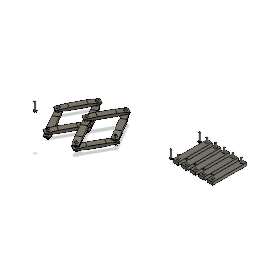
Collapse model encube (Autodesk Fusion 360 design; units mm, degrees)
Autodesk Fusion 360 part; units mm, degrees
sketch "Sketch6" plane through (0, 0, 0) normal (0, 1, 0) x (1, 0, 0)
  line L0 (20, 40) -> (40, 40)
  line L1 (40, 40) -> (40, -80)
  line L2 (40, -80) -> (20, -80)
  line L3 (20, -80) -> (20, 40)
  circle A0 centre (30, -70) radius 5
  circle A1 centre (30, 30) radius 5
  circle A2 centre (30, 30) radius 3.5
  dimension "d15" = 20
  dimension "d16" = 120
  dimension "d17" = 10
  dimension "d18" = 10
  dimension "d19" = 7
  measures "d17" diameter of A0
  measures "d18" diameter of A1
  measures "d19" diameter of A2
extrude "Extrude4" add sketch "Sketch6" along normal blind 10 makes body 1 at (33.4956, 6.6667, -29.8255) makes body 2 at (38.2593, 0, 3.8246)
extrude "Extrude5" add 1 faces at (30.1843, 10, -30.3192) along direction (0, 1, 0) blind 15 on bodies 1 bodies 1
extrude "Extrude6" add 1 faces at (29.8594, 0, -31.0235) along direction (0, -1, 0) blind 2 on bodies 1 bodies 1
sketch "Sketch7" plane through (0, -2, 0) normal (0, -1, 0) x (1, 0, 0)
  circle A0 centre (30, -30) radius 3.5
  circle A1 centre (30, -30) radius 5.5
  dimension "d27" = 11
  measures "d27" diameter of A1
extrude "Extrude7" add sketch "Sketch7" along normal blind 2 contours A0 | A1 bodies 1
copy_body "CopyPasteBodies1" bodies 1 makes body 3
move_body "Move1" bodies 3 to x (1, 0, 0) y (0, 1, 0) z (0, 0, 1) at (0, -1.5, 100)
copy_body "CopyPasteBodies2" bodies 2 3 1 makes body 4 makes body 5 makes body 6
move_body "Move2" bodies 4 5 6 to x (1, 0, 0) y (0, 1, 0) z (0, 0, 1) at (10, -5, 0)
move_body "Move3" bodies 4 5 6 to x (1, 0, 0) y (0, 1, 0) z (0, 0, 1) at (25, 0, 0)
copy_body "CopyPasteBodies3" bodies 6 4 5 makes body 7 makes body 8 makes body 9
move_body "Move4" bodies 7 8 9 to x (1, 0, 0) y (0, 1, 0) z (0, 0, 1) at (10, -5, 0)
move_body "Move5" bodies 4 5 6 to x (1, 0, 0) y (0, 1, 0) z (0, 0, 1) at (-10, 4.9138, 0)
move_body "Move6" bodies 8 7 9 to x (1, 0, 0) y (0, 1, 0) z (0, 0, 1) at (9.3387, 10, 3.5763)
copy_body "CopyPasteBodies4" bodies 9 8 7 makes body 10 makes body 11 makes body 12
move_body "Move7" bodies 10 11 12 to x (1, 0, 0) y (0, 1, 0) z (0, 0, 1) at (30, 0, 0)
copy_body "CopyPasteBodies5" bodies 11 12 10 makes body 13 makes body 14 makes body 15
move_body "Move8" bodies 13 14 15 to x (1, 0, 0) y (0, 1, 0) z (0, 0, 1) at (30, 0, 0)
copy_body "CopyPasteBodies6" bodies 11 12 10 makes body 16 makes body 17 makes body 18
move_body "Move9" bodies 16 17 18 to x (1, 0, 0) y (0, 1, 0) z (0, 0, 1) at (60, 0, 0)
copy_body "CopyPasteBodies7" bodies 11 12 10 makes body 19 makes body 20 makes body 21
move_body "Move10" bodies 19 20 21 to x (1, 0, 0) y (0, 1, 0) z (0, 0, 1) at (-110, 0, 0)
copy_body "CopyPasteBodies8" bodies 11 12 10 makes body 22 makes body 23 makes body 24
move_body "Move11" bodies 22 23 24 to x (1, 0, 0) y (0, 1, 0) z (0, 0, 1) at (90, 0, 0)
move_body "Move12" bodies 19 20 21 to x (0.866025, 0, -0.5) y (0, 1, 0) z (0.5, 0, 0.866025) at (17.4534, 0, -7.7105)
move_body "Move13" bodies 3 1 2 to x (0.866025, 0, 0.5) y (0, 1, 0) z (-0.5, 0, 0.866025) at (35.5324, 0, -103.6086)
move_body "Move14" bodies 3 2 1 to x (1, 0, 0) y (0, 1, 0) z (0, 0, 1) at (-18.3852, 0, -5.657)
move_body "Move15" bodies 20 to x (1, 0, 0) y (0, 1, 0) z (0, 0, 1) at (-36.4098, 0, 16.5628)
move_body "Move16" bodies 2 to x (1, 0, 0) y (0, 1, 0) z (0, 0, 1) at (0, 12, 0)
move_body "Move17" bodies 16 5 6 11 4 23 24 22 12 13 10 18 7 8 14 15 17 9 to x (1, 0, 0) y (0, 1, 0) z (0, 0, 1) at (120, 0, -170)
copy_body "CopyPasteBodies9" bodies 19 2 3 21 1 makes body 25 makes body 26 makes body 27 makes body 28 makes body 29
move_body "Move18" bodies 25 26 27 28 29 to x (-1, 0, 0) y (0, 1, 0) z (0, 0, -1) at (58.6773, 0, -92.8475)
move_body "Move19" bodies 25 27 26 29 28 to x (1, 0, 0) y (0, 1, 0) z (0, 0, 1) at (80, 0, 0)
move_body "Move20" bodies 29 to x (1, 0, 0) y (0, 1, 0) z (0, 0, 1) at (0, 125.2332, 92.6165)
move_body "Move21" bodies 28 to x (1, 0, 0) y (0, 1, 0) z (0, 0, 1) at (0, 145.8501, 251.9169)
move_body "Move22" bodies 27 26 25 to x (0.999848, 0, -0.017452) y (0, 1, 0) z (0.017452, 0, 0.999848) at (-22.4315, -0.8556, 27.9376)
move_body "Move23" bodies 4 to x (1, 0, 0) y (0, 1, 0) z (0, 0, 1) at (-67.9353, -2.2693, 166.4645)
move_body "Move24" bodies 4 to x (0.866025, 0, -0.5) y (0, 1, 0) z (0.5, 0, 0.866025) at (34.7719, 0, 42.6997)
move_body "Move25" bodies 4 to x (1, 0, 0) y (0, 1, 0) z (0, 0, 1) at (17, 0, 0)
move_body "Move26" bodies 4 to x (1, 0, 0) y (0, 1, 0) z (0, 0, 1) at (-20.6603, 15, 6.3397)
move_body "Move27" bodies 4 to x (1, 0, 0) y (0, 1, 0) z (0, 0, 1) at (0, 10, 0)
chamfer "Chamfer1" distance 35 angle 5 1 edges at (102.0647, 32.6444, -42.1957) measured on face at (147.3736, 32.6444, 19.7117) on bodies 4
chamfer "Chamfer2" distance 35 angle 5 1 edges at (102.0647, 22.6444, -42.1957) measured on face at (131.1298, 22.6444, -8.3722) on bodies 4
chamfer "Chamfer3" distance 35 angle 5 2 edges at (111.9128, 21.1444, -42.2817) (111.9128, 11.1444, -42.2817) measured on face at (83.4649, 21.1444, -8.0492) measured on face at (83.4649, 11.1444, -8.0492) on bodies 26
chamfer "Chamfer4" distance 35 angle 5 2 edges at (112.3288, 9.1444, -25.8462) (112.3288, -0.8556, -25.8462) measured on face at (65.9464, 9.1444, -86.9535) measured on face at (65.9464, -0.8556, -86.9535) on bodies 25
chamfer "Chamfer5" distance 35 angle 5 4 edges at (62.9989, 10, 62.4993) (62.9989, 0, 62.4993) (53.7357, 21.1444, 62.6727) (53.7357, 11.1444, 62.6727) measured on face at (33.9579, 10, 28.7686) measured on face at (33.9579, 0, 28.7686) measured on face at (83.5211, 21.1444, 8.6815) measured on face at (83.5211, 11.1444, 8.6815) on bodies 19 26
chamfer "Chamfer6" distance 35 angle 5 4 edges at (2.9989, 10, -41.4237) (2.9989, 0, -41.4237) (3.128, 22, -24.9836) (3.128, 12, -24.9836) measured on face at (33.9378, 10, 11.9148) measured on face at (33.9378, 0, 11.9148) measured on face at (32.169, 22, -58.7143) measured on face at (32.169, 12, -58.7143) on bodies 2 19
chamfer "Chamfer7" distance 35 angle 5 7 edges at (162.0647, 32.6444, 61.7273) (162.0647, 22.6444, 61.7273) (50.5242, 9.1444, -128.7063) (59.0959, 4.1444, -133.8567) (50.5242, -0.8556, -128.7063) (63.128, 22, -128.9066) (63.128, 12, -128.9066) measured on face at (131.3416, 32.6444, 8.2642) measured on face at (131.3416, 22.6444, 8.2642) measured on face at (82.3893, 9.1444, -75.9158) measured on face at (73.6887, 5.8111, -109.5703) measured on face at (82.3893, -0.8556, -75.9158) measured on face at (32.1891, 22, -75.568) measured on face at (32.1891, 12, -75.568) on bodies 2 4 25
move_body "Move28" bodies 21 to x (1, 0, 0) y (0, 1, 0) z (0, 0, 1) at (0, 0, 40)
move_body "Move29" bodies 1 to x (1, 0, 0) y (0, 1, 0) z (0, 0, 1) at (8.3083, 0, -18.1926)
move_body "Move30" bodies 3 to x (1, 0, 0) y (0, 1, 0) z (0, 0, 1) at (-40.9334, 0, -18.6937)
move_body "Move31" bodies 2 to x (0.999391, 0, -0.034899) y (0, 1, 0) z (0.034899, 0, 0.999391) at (2.2194, 0, 1.2079)
move_body "Move32" bodies 1 to x (1, 0, 0) y (0, 1, 0) z (0, 0, 1) at (-5.6261, -6.0621, 8.6157)
move_body "Move33" bodies 1 to x (1, 0, 0) y (0, 1, 0) z (0, 0, 1) at (-5, 0, 9)
move_body "Move34" bodies 1 to x (1, 0, 0) y (0, 1, 0) z (0, 0, 1) at (0.1223, 0, 0.2727)
move_body "Move35" bodies 1 to x (1, 0, 0) y (0, 1, 0) z (0, 0, 1) at (0, 5, 0)
move_body "Move36" bodies 3 to x (1, 0, 0) y (0, 1, 0) z (0, 0, 1) at (41.5864, 0, 19.2805)
extrude "Extrude8" add 1 faces at (106.7267, 22.6444, -32.702) along direction (0, 1, 0) blind 15 on bodies 27 bodies 27
copy_body "CopyPasteBodies10" bodies 26 makes body 30
move_body "Move37" bodies 30 to x (1, 0, 0) y (0, 1, 0) z (0, 0, 1) at (48.481, 0, -87.462)
move_body "Move38" bodies 30 to x (1, 0, 0) y (0, 1, 0) z (0, 0, 1) at (0, 22, 0)
copy_body "CopyPasteBodies11" bodies 26 makes body 31
move_body "Move39" bodies 31 to x (1, 0, 0) y (0, 1, 0) z (0, 0, 1) at (98.5603, 0, -0.7582)
move_body "Move40" bodies 21 to x (1, 0, 0) y (0, 1, 0) z (0, 0, 1) at (0.3864, 0, -39.9909)
move_body "Move41" bodies 28 to x (1, 0, 0) y (0, 1, 0) z (0, 0, 1) at (76.5599, -133.5476, -51.9802)
move_body "Move42" bodies 5 24 18 16 15 12 7 14 10 13 11 23 6 22 17 8 9 to x (1, 0, 0) y (0, 1, 0) z (0, 0, 1) at (160, 0, 0)
copy_body "CopyPasteBodies12" bodies 25 makes body 32
move_body "Move43" bodies 32 to x (0.999962, 0, 0.008727) y (0, 1, 0) z (-0.008727, 0, 0.999962) at (99.3452, 23.0467, -1.5602)
move_body "Move44" bodies 20 to x (1, 0, 0) y (0, 1, 0) z (0, 0, 1) at (234.4691, 9.547, -18.5104)
copy_body "CopyPasteBodies13" bodies 20 makes body 33
move_body "Move45" bodies 33 to x (1, 0, 0) y (0, 1, 0) z (0, 0, 1) at (-50.0211, 12.5, -86.7387)
move_body "Move46" bodies 33 to x (1, 0, 0) y (0, 1, 0) z (0, 0, 1) at (-0.209, 0, 0.3134)
extrude "Extrude9" add 1 faces at (106.7267, 37.6444, -32.702) along direction (0, 1, 0) blind 10 on bodies 27 bodies 27
sketch "Sketch2" plane through (0, 10, 0) normal (0, 1, 0) x (-1, 0, 0)
  line L0 (50, 65) -> (-20, 65)
  line L1 (-20, 65) -> (-20, -25)
  line L2 (-20, -25) -> (50, -25)
  line L3 (50, -25) -> (50, 65)
  circle A0 centre (15, -15) radius 7.0711
sketch "Sketch3" plane through (0, 10, 0) normal (0, 1, 0) x (-1, 0, 0)
  circle A0 centre (15, -15) radius 7.0711
  line L0 (50, 65) -> (-20, 65)
  line L1 (-20, 65) -> (-20, -25)
  line L2 (-20, -25) -> (50, -25)
  line L3 (50, -25) -> (50, 65)
  circle A1 centre (15, -15) radius 6.0711
extrude "Extrude3" [suppressed]
sketch "Sketch5" plane through (0, 0, 0) normal (0, 1, 0) x (1, 0, 0)
  line L0 (46.3278, 25.2078) -> (66.3278, 25.2078)
  line L1 (66.3278, 25.2078) -> (66.3278, -94.7922)
  line L2 (66.3278, -94.7922) -> (46.3278, -94.7922)
  line L3 (46.3278, -94.7922) -> (46.3278, 25.2078)
  circle A0 centre (56.3278, 17.7316) radius 5
  circle A1 centre (56.3278, -86.546) radius 5
  dimension "d11" = 20
  dimension "d12" = 120
  dimension "d13" = 10
  dimension "d14" = 10
  measures "d13" diameter of A0
  measures "d14" diameter of A1
